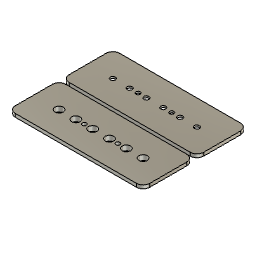
P90-50mm v1 (Autodesk Fusion 360 design; units mm, degrees)
Autodesk Fusion 360 part; units mm, degrees
sketch "スケッチ1" plane through (0, 0, 0) normal (0, 0, 1) x (1, 0, 0)
  line L0 (4, 0) -> (76, 0)
  line L1 (80, 4) -> (80, 26)
  line L2 (76, 30) -> (4, 30)
  line L3 (0, 26) -> (0, 4)
  line L4 (0, 15) -> (80, 15)
  line L5 (40, 30) -> (40, 0)
  line L6 (40, 15) -> (15, 15)
  line L7 (15, 15) -> (25, 15)
  line L8 (25, 15) -> (35, 15)
  line L9 (35, 15) -> (45, 15)
  line L10 (45, 15) -> (55, 15)
  arc A0 (4, 30) -> (0, 26) centre (4, 26) ccw
  arc A1 (80, 26) -> (76, 30) centre (76, 26) ccw
  arc A2 (76, 0) -> (80, 4) centre (76, 4) ccw
  arc A3 (0, 4) -> (4, 0) centre (4, 4) ccw
  point P0 (80, 0)
  point P1 (0, 30)
  point P2 (25, 15)
  point P3 (35, 15)
  point P4 (45, 15)
  point P5 (55, 15)
  point P6 (65, 15)
  dimension "d1" = 80
  dimension "d2" = 30
  dimension "d5" = 25
  dimension "d7" = 10
  dimension "d8" = 10
  dimension "d9" = 10
  dimension "d10" = 10
  dimension "d13" = 4
  constraint horizontal L0
  constraint vertical L1
  constraint horizontal L2
  constraint vertical L3
  constraint midpoint L4 L6.start
  constraint perpendicular L5 L6
  constraint parallel L4 L7
  constraint parallel L4 L8
  constraint parallel L4 L9
  constraint parallel L4 L10
  constraint coincident L2 L5.start
  constraint coincident L3 L4.start
  constraint coincident P1 L2
  constraint coincident P1 L3
  constraint tangent L2 A0
  constraint tangent L3 A0
  constraint coincident L1 L4.end
  constraint tangent L1 A1
  constraint tangent L2 A1
  constraint equal A0 A1
  constraint coincident L0 L5.end
  constraint coincident P0 L0
  constraint coincident P0 L1
  constraint tangent L0 A2
  constraint tangent L1 A2
  constraint equal A0 A2
  constraint coincident origin L0
  constraint coincident origin L3
  constraint tangent L0 A3
  constraint tangent L3 A3
  constraint equal A0 A3
  constraint coincident P2 L7.end
  constraint coincident P4 L9.end
  constraint coincident P5 L10.end
  measures "d1" distance of origin P0
  measures "d2" distance of origin P1
  measures "d5" distance of L6.start L6.end
  measures "d7" distance of L6.end P2
  measures "d8" distance of P2 P3
  measures "d9" distance of P3 P4
  measures "d10" distance of P4 P5
  measures "d13" radius of A0
extrude "押し出し1" add sketch "スケッチ1" along normal blind 2 makes body 1
sketch "スケッチ2" plane through (0, 0, 2) normal (0, 0, 1) x (-1, 0, 0)
  arc A0 (0, -4) -> (-4, 0) centre (-4, -4) ccw
  line L0 (-4, 0) -> (-76, 0)
  arc A1 (-76, 0) -> (-80, -4) centre (-76, -4) ccw
  line L1 (-80, -4) -> (-80, -26)
  arc A2 (-80, -26) -> (-76, -30) centre (-76, -26) ccw
  line L2 (-76, -30) -> (-4, -30)
  arc A3 (-4, -30) -> (0, -26) centre (-4, -26) ccw
  line L3 (0, -26) -> (0, -4)
  line L4 (0, -15) -> (-80, -15)
  point P0 (-45, -15)
  point P1 (-55, -15)
  point P2 (-65, -15)
  point P3 (-35, -15)
  point P4 (-25, -15)
  point P5 (-15, -15)
  constraint midpoint L3 L4.start
  constraint midpoint L1 L4.end
  constraint coincident L4 P0
  constraint coincident L4 P1
  constraint coincident L4 P2
  constraint coincident L4 P3
  constraint coincident L4 P4
  constraint coincident L4 P5
hole "穴2" at (15, 15, 2) at (25, 15, 2) at (35, 15, 2) at (55, 15, 2) at (65, 15, 2) at (45, 15, 2) direction (0, 0, -1) diameter 3 depth 2 tip angle 118 bodies 1
sketch "スケッチ3" plane through (0, 0, 0) normal (0, 0, -1) x (1, 0, 0)
  circle A0 centre (65, -15) radius 1.5
  circle A1 centre (35, -15) radius 1.5
  circle A2 centre (15, -15) radius 1.5
  circle A3 centre (25, -15) radius 1.5
  circle A4 centre (55, -15) radius 1.5
  circle A5 centre (45, -15) radius 1.5
  arc A6 (4, 0) -> (0, -4) centre (4, -4) ccw
  line L0 (0, -4) -> (0, -26)
  arc A7 (0, -26) -> (4, -30) centre (4, -26) ccw
  line L1 (4, -30) -> (76, -30)
  arc A8 (76, -30) -> (80, -26) centre (76, -26) ccw
  line L2 (80, -26) -> (80, -4)
  arc A9 (80, -4) -> (76, 0) centre (76, -4) ccw
  line L3 (76, 0) -> (4, 0)
  line L4 (66.5, -15) -> (68.5, -15)
  line L5 (11.5, -11.5) -> (65, -11.5)
  line L6 (65, -18.5) -> (15, -18.5)
  line L7 (11.5, -15) -> (11.5, -11.5)
  arc A10 (11.5, -15) -> (15, -18.5) centre (15, -15) ccw
  arc A11 (15, -11.5) -> (11.5, -15) centre (15, -15) ccw
  arc A12 (65, -18.5) -> (68.5, -15) centre (65, -15) ccw
  arc A13 (68.5, -15) -> (65, -11.5) centre (65, -15) ccw
  point P0 (11.5, -18.5)
  dimension "d23" = 2
  dimension "d25" = 7
  dimension "d26" = 3.5
  dimension "d27" = 3.5
  constraint coincident A0 L4.start
  constraint parallel L3 L4
  constraint horizontal L5
  constraint horizontal L6
  constraint vertical L7
  constraint coincident P0 L6
  constraint coincident P0 L7
  constraint tangent L6 A10
  constraint tangent L7 A10
  constraint equal A10 A11
  constraint tangent L6 A12
  constraint tangent L5 A13
  constraint equal A12 A13
  constraint coincident L4.end A12.end
  measures "d23" distance of L4.start L4.end
  measures "d25" distance of L5.start P0
  measures "d26" radius of A10
  measures "d27" radius of A12
extrude "押し出し2" cut sketch "スケッチ3" against normal blind 1 contours L5 L6 A10 A11 A12 A13 bodies 1
copy_body "ボディのコピーと貼り付け1" bodies 1 makes body 2
copy_body "ボディのコピーと貼り付け2" bodies 1 makes body 3
copy_body "ボディのコピーと貼り付け3" bodies 2 3 1 makes body 4 makes body 5 makes body 6
move_body "移動1" bodies 4 5 6 to x (1, 0, 0) y (0, 1, 0) z (0, 0, 1) at (0, -32, 0)
sketch "スケッチ4" plane through (0, 0, 1) normal (0, 0, -1) x (1, 0, 0)
  circle A0 centre (35, 17) radius 1.5
  circle A1 centre (25, 17) radius 1.5
  circle A2 centre (15, 17) radius 1.5
  circle A3 centre (55, 17) radius 1.5
  circle A4 centre (45, 17) radius 1.5
  circle A5 centre (65, 17) radius 1.5
  arc A6 (65, 13.5) -> (65, 20.5) centre (65, 17) ccw
  line L0 (65, 20.5) -> (15, 20.5)
  arc A7 (15, 20.5) -> (15, 13.5) centre (15, 17) ccw
  line L1 (15, 13.5) -> (65, 13.5)
extrude "押し出し3" add sketch "スケッチ4" along normal blind 9 bodies 4 5 6
sketch "スケッチ5" plane through (0, 0, 2) normal (0, 0, 1) x (-1, 0, 0)
  circle A0 centre (-65, 17) radius 1.5
  circle A1 centre (-35, 17) radius 1.5
  circle A2 centre (-15, 17) radius 1.5
  circle A3 centre (-25, 17) radius 1.5
  circle A4 centre (-55, 17) radius 1.5
  circle A5 centre (-45, 17) radius 1.5
  arc A6 (0, 28) -> (-4, 32) centre (-4, 28) ccw
  line L0 (-4, 32) -> (-76, 32)
  arc A7 (-76, 32) -> (-80, 28) centre (-76, 28) ccw
  line L1 (-80, 28) -> (-80, 6)
  arc A8 (-80, 6) -> (-76, 2) centre (-76, 6) ccw
  line L2 (-76, 2) -> (-4, 2)
  arc A9 (-4, 2) -> (0, 6) centre (-4, 6) ccw
  line L3 (0, 6) -> (0, 28)
  point P0 (-15, 17)
  point P1 (-25, 17)
  point P2 (-35, 17)
  point P3 (-45, 17)
  point P4 (-55, 17)
  point P5 (-65, 17)
  constraint coincident P0 A2.centre
  constraint coincident P1 A3.centre
  constraint coincident A1.centre P2
  constraint coincident P3 A5.centre
  constraint coincident P4 A4.centre
  constraint coincident P5 A0.centre
hole "穴3" at (55, -17, 2) at (65, -17, 2) at (45, -17, 2) at (35, -17, 2) at (25, -17, 2) at (15, -17, 2) direction (0, 0, -1) diameter 3 depth 10 tip angle 180 counterbore diameter 5 counterbore depth 3 bodies 4
sketch "スケッチ6" plane through (0, 0, 2) normal (0, 0, 1) x (-1, 0, 0)
  circle A0 centre (-65, -15) radius 1.5
  circle A1 centre (-35, -15) radius 1.5
  circle A2 centre (-15, -15) radius 1.5
  circle A3 centre (-25, -15) radius 1.5
  circle A4 centre (-55, -15) radius 1.5
  circle A5 centre (-45, -15) radius 1.5
  arc A6 (0, -4) -> (-4, 0) centre (-4, -4) ccw
  line L0 (-4, 0) -> (-76, 0)
  arc A7 (-76, 0) -> (-80, -4) centre (-76, -4) ccw
  line L1 (-80, -4) -> (-80, -26)
  arc A8 (-80, -26) -> (-76, -30) centre (-76, -26) ccw
  line L2 (-76, -30) -> (-4, -30)
  arc A9 (-4, -30) -> (0, -26) centre (-4, -26) ccw
  line L3 (0, -26) -> (0, -4)
  point P0 (-30, 17)
  point P1 (-50, 17)
  point P2 (-50, -15)
  point P3 (-30, -15)
hole "穴4" at (30, -17, 2) at (50, -17, 2) direction (0, 0, -1) diameter 2.5 depth 10 tip angle 180 bodies 4
sketch "スケッチ7" plane through (0, 0, 2) normal (0, 0, 1) x (-1, 0, 0)
  circle A0 centre (-65, -15) radius 1.5
  circle A1 centre (-35, -15) radius 1.5
  circle A2 centre (-15, -15) radius 1.5
  circle A3 centre (-25, -15) radius 1.5
  circle A4 centre (-55, -15) radius 1.5
  circle A5 centre (-45, -15) radius 1.5
  arc A6 (0, -4) -> (-4, 0) centre (-4, -4) ccw
  line L0 (-4, 0) -> (-76, 0)
  arc A7 (-76, 0) -> (-80, -4) centre (-76, -4) ccw
  line L1 (-80, -4) -> (-80, -26)
  arc A8 (-80, -26) -> (-76, -30) centre (-76, -26) ccw
  line L2 (-76, -30) -> (-4, -30)
  arc A9 (-4, -30) -> (0, -26) centre (-4, -26) ccw
  line L3 (0, -26) -> (0, -4)
  point P0 (-30, -15)
  point P1 (-50, -15)
hole "穴5" at (30, 15, 2) at (50, 15, 2) direction (0, 0, -1) diameter 2.5 depth 1 tip angle 180 bodies 1 2 3
